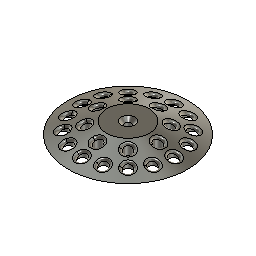
TinVesselHolderV5 (Autodesk Fusion 360 design; units mm, degrees)
Autodesk Fusion 360 part; units mm, degrees
sketch "Sketch2" plane through (0, 0, 0) normal (1, 0, 0) x (0, 1, 0) in component "BasePlate"
  line L0 (0, 0) -> (50, 0)
  line L1 (50, 0) -> (17.75, 10)
  line L2 (17.75, 10) -> (2.75, 10)
  line L3 (2.75, 10) -> (2.75, 3)
  line L4 (2.75, 3) -> (0, 3)
  line L5 (0, 3) -> (0, 0)
  dimension "d7" = 3
  dimension "d8" = 2.75
  dimension "d9" = 7
  dimension "d10" = 15
  dimension "d11" = 50
  constraint coincident L0.start L5.end
  constraint horizontal L0
  constraint parallel L0 L2
  constraint perpendicular L2 L3
  constraint perpendicular L3 L4
  constraint perpendicular L0 L5
  measures "d7" distance of L0 L4
  measures "d8" distance of L3 L5
  measures "d9" distance of L2 L4
  measures "d10" distance of L1.end L2.end
  measures "d11" distance of L0.start L0.end
revolve "Revolve3" add sketch "Sketch2" angle 360 about axis through (0, 0, 1.75) along (0, 0, 1) in component "BasePlate"
sketch "Sketch6" plane through (0, 0, 0) normal (0, 0, -1) x (1, 0, 0) in component "BasePlate"
  circle A0 centre (0, 0) radius 50
  circle A1 centre (0, -38) radius 3.5
  circle A2 centre (0, -25) radius 3.5
  circle A3 centre (14.542, -35.1074) radius 3.5
  circle A4 centre (26.8701, -26.8701) radius 3.5
  circle A5 centre (35.1074, -14.542) radius 3.5
  circle A6 centre (38, 0) radius 3.5
  circle A7 centre (35.1074, 14.542) radius 3.5
  circle A8 centre (26.8701, 26.8701) radius 3.5
  circle A9 centre (14.542, 35.1074) radius 3.5
  circle A10 centre (0, 38) radius 3.5
  circle A11 centre (-14.542, 35.1074) radius 3.5
  circle A12 centre (-26.8701, 26.8701) radius 3.5
  circle A13 centre (-35.1074, 14.542) radius 3.5
  circle A14 centre (-38, 0) radius 3.5
  circle A15 centre (-35.1074, -14.542) radius 3.5
  circle A16 centre (-26.8701, -26.8701) radius 3.5
  circle A17 centre (-14.542, -35.1074) radius 3.5
  circle A18 centre (17.6777, -17.6777) radius 3.5
  circle A19 centre (25, 0) radius 3.5
  circle A20 centre (17.6777, 17.6777) radius 3.5
  circle A21 centre (0, 25) radius 3.5
  circle A22 centre (-17.6777, 17.6777) radius 3.5
  circle A23 centre (-25, 0) radius 3.5
  circle A24 centre (-17.6777, -17.6777) radius 3.5
  dimension "d35" = 7
  dimension "d36" = 7
  dimension "d37" = 25
  dimension "d38" = 38
  dimension "d40" = 360
  dimension "d42" = 360
  measures "d35" diameter of A1
  measures "d36" diameter of A2
  measures "d37" distance of A0.centre A2.centre
  measures "d38" distance of A0.centre A1.centre
extrude "Extrude4" cut sketch "Sketch6" along normal up to surface contours A1 | A2 | A3 | A4 | A5 | A6 | A7 | A8 | A9 | A10 | A11 | A12 | A13 | A14 | A15 | A16 | A17 | A18 | A19 | A20 | A21 | A22 | A23 | A24 end surface at (39.8724, -15.6488, 2.2222) in component "BasePlate"
chamfer "Chamfer3" distance 3 angle 45 1 edges at (-2.5639, 0.9944, 10) in component "BasePlate"
fillet "Fillet1" radius 2 24 edges at (-17.8838, 34.0703, 3.5725) (-29.5606, 24.6331, 3.5725) (-36.7371, 11.4456, 3.5725) (-38.3207, -3.4843, 3.5725) (-34.0703, -17.8838, 3.5725) (-24.6331, -29.5606, 3.5725) (-11.4456, -36.7371, 3.5725) (3.4843, -38.3207, 3.5725) (17.8838, -34.0703, 3.5725) (29.5606, -24.6331, 3.5725) (3.464, -25.495, 7.5258) (-15.5783, -20.4771, 7.5258) (-25.495, -3.464, 7.5258) (-20.4771, 15.5783, 7.5258) (-3.464, 25.495, 7.5258) (-3.4843, 38.3207, 3.5725) (11.4456, 36.7371, 3.5725) (15.5783, 20.4771, 7.5258) (24.6331, 29.5606, 3.5725) (34.0703, 17.8838, 3.5725) (38.3207, 3.4843, 3.5725) (36.7371, -11.4456, 3.5725) (25.495, 3.464, 7.5258) (20.4771, -15.5783, 7.5258) in component "BasePlate"
component "BasePlate" placed x (1, 0, 0) y (0, 1, 0) z (0, 0, 1) at (0, 0, 0)
equation "d8 = ( 5.5 / 2 ) * 1 mm"
